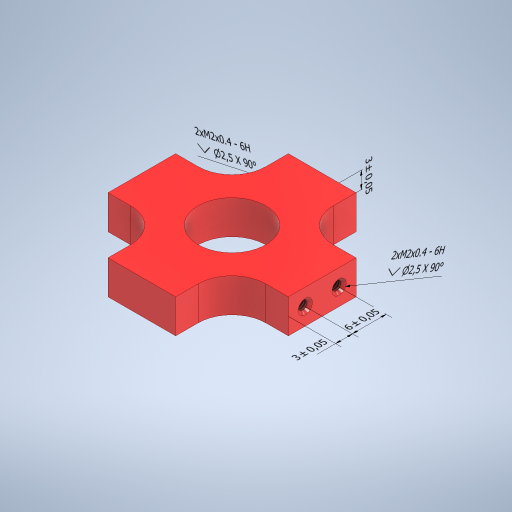
# Autodesk Inventor part: rapoukMiddleLeg0v3
Saved by Autodesk Inventor 2024 (Build 280153000, 153)
## iProperties
Created: 2023-05-29
Part Number: rapoukMiddleLeg0v3
Material: EN AW-6060 T6
Document SubType Name: Modeling
Designer: Roman
Density: 2.7 g/cm^3
Appearance: Light Red
Mass: 8.21344 g
Surface Area: 24.2498 cm^2
Volume: 3.04202 cm^3
Description: Kříž nohy
Polotovar: KR...
Author: Roman
Autodesk Inventor part; units mm, degrees
ref_plane "YZ Plane" through (0, 0, 0) normal (1, 0, 0) x (0, 1, 0)
ref_plane "XZ Plane" through (0, 0, 0) normal (0, 1, 0) x (-1, 0, 0)
ref_plane "XY Plane" through (0, 0, 0) normal (0, 0, 1) x (1, 0, 0)
sketch "Sketch1" plane through (0, 0, 0) normal (0, 1, 0) x (-1, 0, 0)
  line L0 (-6, 6) -> (6, 6)
  line L1 (6, 6) -> (6, -6)
  line L2 (6, -6) -> (-6, -6)
  line L3 (-6, -6) -> (-6, 6)
  line L4 (-6, 6) -> (6, -6) construction
  line L5 (6, 6) -> (-6, -6) construction
  line L6 (6, 6) -> (16, 6)
  line L7 (16, -6) -> (6, -6)
  line L8 (6, -6) -> (6, 6)
  line L9 (0, 6) -> (0, -6) construction
  line L10 (-6, 6) -> (-16, 6)
  line L11 (-16, 6) -> (-16, -6)
  line L12 (-16, -6) -> (-6, -6)
  line L13 (-6, -6) -> (-6, -16)
  line L14 (-6, -16) -> (6, -16)
  line L15 (6, -16) -> (6, -6)
  line L16 (6, 6) -> (6, 16)
  line L17 (6, 16) -> (-6, 16)
  line L18 (-6, 16) -> (-6, 6)
  line L19 (16, 6) -> (16, -6)
  line L20 (6, 6) -> (-6, -6) construction
  line L21 (-6, 6) -> (6, -6) construction
  line L22 (-6, -6) -> (6, 6) construction
  circle A0 centre (0, 0) radius 6
  dimension "d0" = 12
  dimension "d1" = 12
  dimension "d6" = 12
  dimension "d38" = 12
  dimension "d39" = 10
  dimension "d40" = 10
  constraints: 46 end point, 14 symmetric about line, 4 midpoint, 3 parallel, 2 horizontal, 1 centre point, 1 coincident, 1 perpendicular
  measures "d0" distance of L1.end L2.end
  measures "d1" distance of L0.end L1.end
  measures "d6" diameter of A0
  measures "d38" distance between parallel lines of L7 L6
  measures "d39" distance between parallel lines of L14 L2
  measures "d40" distance between parallel lines of L19 L8
extrude "Extrusion9" add sketch "Sketch1" along normal blind 6 contours L18 L17 L16 L0 | L0 A0 L3 | L3 L12 L11 L10 | L0 L1 A0 | A0 L2 L3 | L6 L19 L7 L1 | L1 L2 A0 | L2 L15 L14 L13
fillet "Fillet4" radius 6 4 edges at (-6, 3, -6) (6, 3, -6) (-6, 3, 6) (6, 3, 6)
sketch "Sketch11" plane through (16, 0, 6) normal (1, 0, 0) x (0, 0, -1)
  line L0 (6, 0) -> (6, 6)
  line L1 (0, 6) -> (12, 6) projected
  circle A0 centre (9, 3) radius 1
  line L2 (12, 0) -> (12, 6) projected
  line L3 (0, 0) -> (12, 0) projected
  circle A1 centre (3, 3) radius 1
  dimension "d69" = 2
  dimension "d70" = 3
  dimension "d71" = 3
  constraints: 2 centre point, 2 end point, 1 midpoint, 1 symmetric about line, 1 other
  measures "d69" diameter of A0
  measures "d70" distance from line of L2 A0.centre
  measures "d71" distance from line of L3 A0.centre
hole "Hole1" at (16, 3, 3) at (16, 3, -3) direction (-1, 0, 0) diameter 1.567 depth 6.3 tip angle 118 countersink diameter 2.5 countersink angle 90 thread size "M2x0.4" class "6H" standard "ISO Metric profile"
sketch "Sketch14" plane through (6, 0, -16) normal (0, 0, -1) x (-1, 0, 0)
  line L0 (6, 0) -> (6, 6)
  line L1 (0, 6) -> (12, 6) projected
  circle A0 centre (9, 3) radius 1
  line L2 (12, 0) -> (12, 6) projected
  line L3 (0, 0) -> (12, 0) projected
  circle A1 centre (3, 3) radius 1
  dimension "d99" = 2
  dimension "d100" = 3
  dimension "d101" = 3
  constraints: 2 centre point, 2 end point, 1 midpoint, 1 symmetric about line, 1 other
  measures "d99" diameter of A0
  measures "d100" distance from line of L2 A0.centre
  measures "d101" distance from line of L3 A0.centre
hole "Hole2" at (3, 3, -16) at (-3, 3, -16) direction (0, 0, 1) diameter 1.567 depth 6.3 tip angle 118 countersink diameter 2.5 countersink angle 90 thread size "M2x0.4" class "6H" standard "ISO Metric profile"
body "Solid2"
